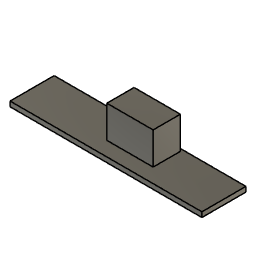
Curtains Cap (Autodesk Fusion 360 design; units mm, degrees)
Autodesk Fusion 360 part; units mm, degrees
sketch "Sketch1" plane through (0, 0, 0) normal (0, 0, 1) x (1, 0, 0)
  line L0 (77.5, 0) -> (77.5, 17.8)
  line L1 (0, 17.8) -> (0, 0)
  line L2 (52, 5.8) -> (52, 16.8)
  line L3 (52, 16.8) -> (33.3, 16.8)
  line L4 (33.3, 16.8) -> (33.3, 5.8)
  line L5 (77.5, 17.8) -> (62.1, 17.8)
  line L6 (58.4, 17.8) -> (26.9, 17.8)
  line L7 (23.2, 17.8) -> (0, 17.8)
  line L8 (0, 0) -> (39.3, 0)
  line L9 (46, 0) -> (77.5, 0)
  line L10 (33.3, 5.8) -> (39.3, 5.8)
  line L11 (46, 5.8) -> (52, 5.8)
  line L12 (39.3, 5.8) -> (46, 5.8)
  line L13 (39.3, 0) -> (46, 0)
  line L14 (62.1, 17.8) -> (58.4, 17.8)
  line L15 (23.2, 17.8) -> (26.9, 17.8)
  dimension "d1" = 77.5
  dimension "d2" = 17.8
  dimension "d25" = 11
  dimension "d26" = 1
  constraint horizontal L8
  constraint vertical L0
  constraint horizontal L5
  constraint vertical L1
  constraint coincident L1.end L8.start
  constraint coincident L6.start L5
  constraint coincident L7.start L5
  constraint coincident L6.end L5
  constraint horizontal L10
  constraint vertical L2
  constraint horizontal L3
  constraint vertical L4
  constraint collinear L5 L6
  constraint collinear L6 L7
  constraint coincident L11.start L10
  constraint coincident L9.start L8
  constraint collinear L8 L9
  constraint collinear L10 L11
  constraint horizontal L15
  measures "d1" distance of L1.end L0.start
  measures "d2" distance of L1.end L1.start
  measures "d25" distance of L3 L10
  measures "d26" distance of L3 L5
extrude "Extrude1" add sketch "Sketch1" along normal blind 2
extrude "Extrude2" add sketch "Sketch1" along normal blind 15 contours L2 L3 L4 L10 L11 L12
sketch "Sketch2" plane through (0, 0, 0) normal (0, 0, 1) x (1, 0, 0)
  line L0 (33.3, 5.8) -> (39.3, 5.8)
  line L1 (39.3, 5.8) -> (46, 5.8)
  line L2 (46, 5.8) -> (52, 5.8)
  line L3 (52, 5.8) -> (52, 16.8)
  line L4 (33.3, 16.8) -> (33.3, 5.8)
  line L5 (52, 16.8) -> (33.3, 16.8)
  line L6 (48, 8) -> (37.3, 8)
  line L7 (37.3, 8) -> (37.3, 14.6)
  line L8 (37.3, 14.6) -> (48, 14.6)
  line L9 (48, 14.6) -> (48, 8)
  line L10 (48, 8) -> (37.3, 14.6) construction
  line L11 (37.3, 8) -> (48, 14.6) construction
  point P0 (42.65, 11.3)
  constraint horizontal L6
  constraint perpendicular L6 L7
  constraint parallel L6 L8
  constraint parallel L7 L9
  constraint coincident L10 P0
  constraint coincident L11 P0
